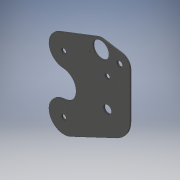
# Autodesk Inventor part: Shooter Side Plate
Saved by Autodesk Inventor 2019.4 (Build 234330000, 330)
## iProperties
Created: 2020-01-16
Part Number: Shooter Side Plate
Material: CFRP
Document SubType Name: Modeling
Designer: admin
Density: 1.43 g/cm^3
Appearance: Carbon Fiber
Mass: 646.666 g
Surface Area: 1906.29 cm^2
Volume: 452.214 cm^3
Author: admin
Autodesk Inventor part; units mm, degrees
ref_plane "YZ Plane" through (0, 0, 0) normal (1, 0, 0) x (0, 1, 0)
ref_plane "XZ Plane" through (0, 0, 0) normal (0, 1, 0) x (-1, 0, 0)
ref_plane "XY Plane" through (0, 0, 0) normal (0, 0, 1) x (1, 0, 0)
sketch "Sketch1" plane through (0, 0, 0) normal (0, 0, 1) x (1, 0, 0)
  arc A0 (88.9, 0) -> (37.9634, -80.3865) centre (0, 0) ccw construction
  circle A1 centre (0, 114.3) radius 50.8 construction
  circle A2 centre (-174.3511, 114.3) radius 50.8 construction
  circle A3 centre (-174.3511, -114.3) radius 50.8 construction
  line L0 (-174.3511, 114.3) -> (-174.3511, -114.3) construction
  line L1 (-174.3511, 0) -> (0, 0) construction
  circle A4 centre (-174.3511, -114.3) radius 9.5
  circle A5 centre (-174.3511, 114.3) radius 9.5
  circle A6 centre (0, 114.3) radius 9.5
  line L2 (0, 0) -> (0, 114.3) construction
  circle A7 centre (-26.7764, 192.7449) radius 11
  circle A8 centre (48.9, 181.2281) radius 11
  line L3 (0, 114.3) -> (48.9, 181.2281) construction
  line L4 (0, 114.3) -> (-26.7764, 192.7449) construction
  circle A9 centre (48.9, 181.2281) radius 32.5 construction
  circle A10 centre (-26.7764, 192.7449) radius 32.5
  line L5 (0, 0) -> (-490.9821, 0) construction
  arc A11 (54.9181, 220.7728) -> (88.9, 181.2281) centre (48.9, 181.2281) ccw construction
  line L6 (88.9, 181.2281) -> (88.9, 0)
  arc A12 (-41.1896, 230.058) -> (-20.7583, 232.2896) centre (-26.7764, 192.7449) ccw construction
  line L7 (-20.7583, 232.2896) -> (54.9181, 220.7728)
  arc A13 (-195.9708, 170.2695) -> (-177.3128, 54.3731) centre (-174.3511, 114.3) ccw
  arc A14 (-177.3128, -54.3731) -> (-148.7289, -168.5541) centre (-174.3511, -114.3) ccw
  line L8 (-195.9708, 170.2695) -> (-41.1896, 230.058)
  line L9 (-148.7289, -168.5541) -> (37.9634, -80.3865)
  arc A15 (-177.3128, -54.3731) -> (-177.3128, 54.3731) centre (-180, 0) ccw
  arc A16 (37.9634, -80.3865) -> (88.9, 0) centre (0, 0) ccw
  arc A17 (88.9, 181.2281) -> (54.9181, 220.7728) centre (48.9, 181.2281) ccw
  arc A18 (-20.7583, 232.2896) -> (-41.1896, 230.058) centre (-26.7764, 192.7449) ccw
  arc A19 (-177.3128, 54.3731) -> (-195.9708, 170.2695) centre (-174.3511, 114.3) ccw construction
  arc A20 (-148.7289, -168.5541) -> (-177.3128, -54.3731) centre (-174.3511, -114.3) ccw construction
  circle A21 centre (0, 0) radius 16
  line L10 (-174.3511, -114.3) -> (0, 114.3) construction
  dimension "d37" = 177.8
  dimension "d38" = 101.6
  dimension "d39" = 101.6
  dimension "d40" = 101.6
  dimension "d41" = 19
  dimension "d42" = 19
  dimension "d43" = 19
  dimension "d44" = 114.3
  dimension "d46" = 228.6
  dimension "d47" = 22
  dimension "d48" = 22
  dimension "d49" = 82.889
  dimension "d50" = 65
  dimension "d51" = 82.889
  dimension "d52" = 65
  dimension "d53" = 55
  dimension "d54" = 0
  dimension "d55" = 174.351
  dimension "d56" = 80
  dimension "d57" = 80
  dimension "d58" = 120
  dimension "d59" = 120
  dimension "d60" = 180
  dimension "d61" = 32
  dimension "d64" = 287.5
  constraints: 22 centre point, 22 end point, 22 point on circle, 11 coincident, 9 tangent, 2 perpendicular, 1 horizontal, 1 midpoint, 1 parallel, 1 point on line
  measures "d37" diameter of A0
  measures "d38" diameter of A1
  measures "d39" diameter of A2
  measures "d40" diameter of A3
  measures "d41" diameter of A4
  measures "d42" diameter of A5
  measures "d43" diameter of A6
  measures "d44" distance of L1.end L2.end
  measures "d46" distance of L0.start L0.end
  measures "d47" diameter of A7
  measures "d48" diameter of A8
  measures "d49" distance of L2.end L3.end
  measures "d50" diameter of A9
  measures "d51" distance of L2.end L4.end
  measures "d52" diameter of A10
  measures "d53" angle of L3 L4
  measures "d54" distance between parallel lines of L1 L5
  measures "d55" distance from line of point (0, 0) L0
  measures "d56" diameter of A11
  measures "d57" diameter of A12
  measures "d58" diameter of A13
  measures "d59" diameter of A14
  measures "d60" distance of point (0, 0) A15.centre
  measures "d61" diameter of A21
  measures "d64" distance of L10.start L2.end
extrude "Extrusion1" add sketch "Sketch1" along normal blind 5 contours L6 A16 L9 A14 A15 A13 L8 A18 L7 A17
sketch "Sketch2" plane through (0, 0, 5) normal (0, 0, 1) x (1, 0, 0)
  circle A0 centre (15.6775, 219.1583) radius 2.75 projected
  circle A1 centre (-69.2303, 166.3316) radius 2.75 projected
  point P0 (0, 0)
extrude "Extrusion2" cut sketch "Sketch2" against normal through all
body "Solid1"
